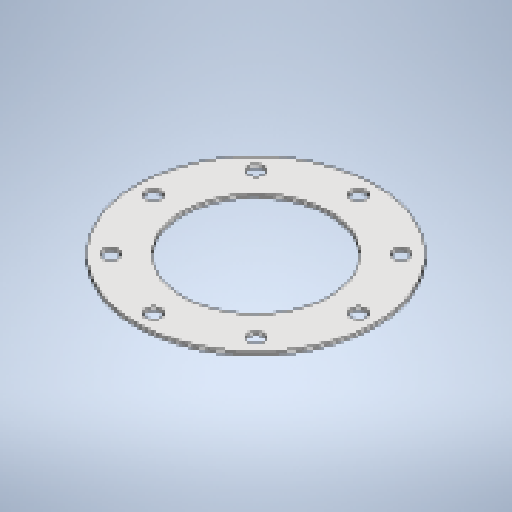
# Autodesk Inventor part: DSB 112 drain system loose flange
Saved by Autodesk Inventor 2025.1 (Build 291241020, 241B)
## iProperties
Created: 2024-12-09
Part Number: DSB 112 drain system loose flange
Material: Stainless Steel
Document SubType Name: Sheet Metal
Designer: user
Mass: 1674.72 g
Surface Area: 927.524 cm^2
Volume: 209.34 cm^3
Density: 8 g/cm^3
Flat Pattern Width: 28 cm
Flat Pattern Length: 28 cm
Flat Pattern Area: 784 cm^2
Sheet Metal Rule: AISI304 4mm Die 32
Sheet Metal Width: 280.000 mm
Sheet Metal Length: 280.000 mm
Sheet Metal Area: 78400.000 mm^2
Appearance: Default
Octaeder_side: 55.919 mm
Octaeder_flange_lenth: 72.500 mm
Author: user
Autodesk Inventor part; units mm, degrees
ref_plane "YZ Plane" through (0, 0, 0) normal (1, 0, 0) x (0, 1, 0)
ref_plane "XZ Plane" through (0, 0, 0) normal (0, 1, 0) x (-1, 0, 0)
ref_plane "XY Plane" through (0, 0, 0) normal (0, 0, 1) x (1, 0, 0)
sketch "Sketch1" plane through (0, 0, 0) normal (0, 0, 1) x (1, 0, 0)
  circle A0 centre (0, 0) radius 86
  circle A1 centre (0, 0) radius 140
  line L0 (98.9949, -98.9949) -> (-98.9949, 98.9949) construction
  line L1 (-98.9949, -98.9949) -> (98.9949, 98.9949) construction
  point P0 (0, 86)
  dimension "d44" = 172
  dimension "d23" = 280
  measures "d23" diameter of A1
extrude "Plate1" add sketch "Sketch1" along normal blind 4
sketch "Sketch6" plane through (0, 0, 0) normal (0, 0, 1) x (1, 0, 0)
  line L0 (0, 0) -> (0, 120) construction
  circle A0 centre (0, 0) radius 120 construction
  line L1 (0, 0) -> (84.8528, 84.8528) construction
  circle A1 centre (84.8528, 84.8528) radius 9
  dimension "d32" = 18
  dimension "d33" = 240
  dimension "d34" = 45
  constraints: 4 end point, 2 centre point, 2 coincident, 2 point on circle, 1 vertical
  measures "d32" diameter of A1
  measures "d33" diameter of A0
  measures "d34" angle of L0 L1
extrude "Cut2" cut sketch "Sketch6" along normal blind 4
pattern_circular "Circular Pattern2" count 8 over 360 about axis through (0, 0, -10) along (0, 0, -1) of "Cut2"
equation "\"d23\" = Flange_D_outer"
equation "\"d32\" = Flange_d_hole_diam"
equation "\"d33\" = Flange_D1_hole_center"
equation "\"d35\" = Thickness"
equation "\"d2\" = Thickness"
equation "\"BendReliefWidth\" = Thickness"
equation "\"BendReliefDepth\" = 0.5 * Thickness"
equation "\"CornerReliefSize\" = 4 * Thickness"
equation "\"MinimumRemnant\" = 2 * Thickness"
equation "\"TransitionRadius\" = BendRadius"
equation "\"JacobiRadiusSize\" = BendRadius"
equation "\"GapSize\" = Thickness"
equation "\"Octaeder_side\" = d41"
equation "\"Octaeder_flange_lenth\" = d42"
equation "\"Flange_D_outer\" = 280"
equation "\"Flange_d_hole_diam\" = 18"
equation "\"Flange_D1_hole_center\" = 240"
equation "\"Thickness\" = 4"
equation "\"BendRadius\" = 6"
equation "\"d41\" = 55.918831"
equation "\"d42\" = 72.5"
body "Solid1"
